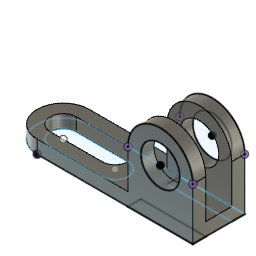
Exercise 5 v0 (Autodesk Fusion 360 design; units mm, degrees)
Autodesk Fusion 360 part; units mm, degrees
sketch "Sketch1" plane through (0, 0, 0) normal (0, 0, 1) x (1, 0, 0)
  line L0 (0, 0) -> (120, 0)
  line L1 (120, 0) -> (120, 40)
  line L2 (120, 40) -> (0, 40)
  arc A0 (0, 40) -> (0, 0) centre (0, 20) ccw
  line L3 (120, 40) -> (70, 40)
  line L4 (70, 40) -> (70, 30)
  line L5 (70, 30) -> (120, 30)
  line L6 (120, 30) -> (120, 40)
  line L7 (120, 0) -> (70, 0)
  line L8 (70, 0) -> (70, 10)
  line L9 (70, 10) -> (120, 10)
  line L10 (120, 10) -> (120, 0)
  line L11 (0, 30) -> (40, 30)
  line L12 (0, 10) -> (40, 10)
  arc A1 (0, 30) -> (0, 10) centre (0, 20) ccw
  arc A2 (40, 10) -> (40, 30) centre (40, 20) ccw
  dimension "d1" = 120
  dimension "d2" = 40
  dimension "d3" = 50
  dimension "d4" = 10
  dimension "d5" = 50
  dimension "d6" = 10
  dimension "d7" = 20
  dimension "d8" = 40
  dimension "d9" = 20
  constraint horizontal L0
  constraint vertical L1
  constraint horizontal L2
  constraint coincident L0.start A0.end
  constraint horizontal L3
  constraint vertical L4
  constraint horizontal L5
  constraint vertical L6
  constraint horizontal L7
  constraint vertical L8
  constraint horizontal L9
  constraint vertical L10
  constraint concentric A0 A1
  constraint tangent L11 A2
  constraint tangent L12 A2
  measures "d1" distance of L0.start L0.end
  measures "d2" distance of L0.start L2.end
  measures "d3" distance of L1.end L3.end
  measures "d4" distance of L1.end L5.end
  measures "d5" distance of L0.end L7.end
  measures "d6" distance of L0.end L9.end
  measures "d7" diameter of A1
  measures "d8" distance of A0.centre A2.centre
  measures "d9" diameter of A2
extrude "Extrude1" add sketch "Sketch1" along normal blind 10 contours L0 L1 L2 A0 L4 L5 L8 L9
extrude "Extrude2" add sketch "Sketch1" along normal blind 40 contours L0 L1 L7 L8 L9 L10 | L1 L2 L3 L4 L5 L6
sketch "Sketch2" plane through (0, 0, 0) normal (0, -1, 0) x (1, 0, 0)
  line L0 (0, 0) -> (120, 0)
  line L1 (120, 0) -> (120, 40)
  line L2 (120, 40) -> (70, 40)
  line L3 (70, 40) -> (70, 10)
  line L4 (70, 10) -> (0, 10)
  line L5 (0, 10) -> (0, 0)
  circle A0 centre (95, 40) radius 15
  arc A1 (120, 40) -> (70, 40) centre (95, 40) ccw
  dimension "d14" = 30
  dimension "d15" = 50
  constraint midpoint L2 A0.centre
  constraint concentric A0 A1
  measures "d14" diameter of A0
  measures "d15" diameter of A1
extrude "Extrude3" add sketch "Sketch2" against normal blind 10 contours L2 A0 A1
extrude "Extrude4" cut sketch "Sketch2" against normal blind 10 contours L2 A0 picked at (96.1126, 35.1254)
sketch "Sketch3" plane through (0, 40, 0) normal (0, 1, 0) x (-1, 0, 0)
  line L0 (-120, 0) -> (0, 0)
  line L1 (0, 0) -> (0, 10)
  line L2 (0, 10) -> (-70, 10)
  line L3 (-70, 10) -> (-70, 40)
  line L4 (-70, 40) -> (-120, 40)
  line L5 (-120, 40) -> (-120, 0)
  circle A0 centre (-95, 40) radius 15
  arc A1 (-70, 40) -> (-120, 40) centre (-95, 40) ccw
  dimension "d20" = 30
  dimension "d21" = 50
  constraint midpoint L4 A0.centre
  constraint concentric A0 A1
  measures "d20" diameter of A0
  measures "d21" diameter of A1
extrude "Extrude5" cut sketch "Sketch3" against normal blind 10 contours L4 A0 picked at (-93.8874, 35.1254)
extrude "Extrude6" add sketch "Sketch3" against normal blind 10 contours L4 A0 A1
